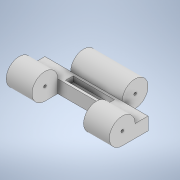
# Autodesk Inventor part: фаланга гусеницы
Saved by Autodesk Inventor 2020.1 (Build 241239000, 239)
## iProperties
Created: 2021-09-27
Part Number: фаланга гусеницы
Material: Типовые
Document SubType Name: Modeling
Designer: User
Density: 1 g/cm^3
Appearance: По умолчанию
Author: User
Autodesk Inventor part; units mm, degrees
ref_plane "YZ Plane" through (0, 0, 0) normal (1, 0, 0) x (0, 1, 0)
ref_plane "XZ Plane" through (0, 0, 0) normal (0, 1, 0) x (-1, 0, 0)
ref_plane "XY Plane" through (0, 0, 0) normal (0, 0, 1) x (1, 0, 0)
sketch "Эскиз1" plane through (0, 0, 0) normal (1, 0, 0) x (0, 1, 0)
  line L0 (0, 0) -> (-5, 0)
  line L1 (-5, 0) -> (-5, -15)
  line L2 (-5, -15) -> (0, -15)
  line L3 (0, -15) -> (0, 0)
  circle A0 centre (0, 0) radius 5
  circle A1 centre (0, -15) radius 5
  circle A2 centre (0, 0) radius 0.5
  circle A3 centre (0, -15) radius 0.5
  point P0 (0, -5)
  point P1 (0, -10)
  dimension "d0" = 5
  dimension "d1" = 15
  dimension "d4" = 1
  dimension "d5" = 1
  constraints: 8 end point, 4 coincident, 2 centre point, 2 parallel, 1 horizontal, 1 perpendicular, 6 other
  measures "d0" distance of L1.end L2.end
  measures "d1" distance of L0.end L1.end
  measures "d4" diameter of A2
  measures "d5" diameter of A3
extrude "Выдавливание1" add sketch "Эскиз1" along normal blind 40 contours A2 L3 A0 L0 | L0 A0 L3 A2 | A0 L3 A1 L1 | A1 L3 A3 L2 | L2 A3 L3 A1
sketch "Эскиз2" plane through (0, 0, -5) normal (0, 1, 0) x (1, 0, 0)
  line L0 (0, 0) -> (40, 0) projected
  line L1 (0, -10) -> (40, -10) projected
  line L2 (10, 0) -> (30, 0)
  line L3 (30, 0) -> (30, -10)
  line L4 (30, -10) -> (10, -10)
  line L5 (10, -10) -> (10, 0)
  line L6 (0, 5) -> (0, 0) projected
  line L7 (40, 5) -> (40, 0) projected
  point P0 (0, -5)
  dimension "d6" = 10
  dimension "d7" = 10
  constraints: 8 end point, 2 parallel, 2 point on line, 1 horizontal, 1 perpendicular
  measures "d6" distance from line of L6 L2.start
  measures "d7" distance from line of L7 L2.end
extrude "Выдавливание2" cut sketch "Эскиз2" along normal mid plane 10
sketch "Эскиз3" plane through (0, 0, -5) normal (0, 1, 0) x (1, 0, 0)
  line L0 (0, 5) -> (40, 5) projected
  line L1 (0, 15) -> (40, 15) projected
  line L2 (10, 5) -> (0, 5)
  line L3 (0, 5) -> (0, 15)
  line L4 (0, 15) -> (10, 15)
  line L5 (10, 15) -> (10, 5)
  line L6 (40, 5) -> (40, 15) projected
  line L7 (30, 5) -> (40, 5)
  line L8 (40, 5) -> (40, 15)
  line L9 (40, 15) -> (30, 15)
  line L10 (30, 15) -> (30, 5)
  line L11 (40, 5) -> (40, 0) projected
  line L12 (0, 5) -> (0, 0) projected
  point P0 (0, -5)
  point P1 (40, 10)
  point P2 (10, 15)
  dimension "d10" = 10
  dimension "d11" = 10
  constraints: 16 end point, 4 parallel, 3 point on line, 2 horizontal, 2 perpendicular
  measures "d10" distance from line of L11 L7.start
  measures "d11" distance from line of L12 L2.start
extrude "Выдавливание3" cut sketch "Эскиз3" against normal mid plane 10 contours L3 L1 L5 L0 | L10 L1 L6 L0
sketch "Эскиз10" plane through (10, 0, -5) normal (0, 1, 0) x (1, 0, 0)
  line L0 (2, 1) -> (18, 1)
  line L1 (18, 1) -> (18, 4)
  line L2 (18, 4) -> (2, 4)
  line L3 (2, 4) -> (2, 1)
  line L4 (20, -10) -> (20, 0) projected
  line L5 (0, 5) -> (0, 15) projected
  line L6 (0, 0) -> (20, 0) projected
  line L7 (-10, 5) -> (0, 5) projected
  point P0 (-10, -5)
  point P1 (20, -5)
  point P2 (0, 10)
  dimension "d37" = 2
  dimension "d38" = 2
  dimension "d39" = 1
  dimension "d40" = 1
  constraints: 8 end point, 2 parallel, 1 horizontal, 1 perpendicular
  measures "d37" distance from line of L4 L0.end
  measures "d38" distance from line of L5 L0.start
  measures "d39" distance from line of L6 L0.start
  measures "d40" distance from line of L7 L2.end
extrude "Выдавливание9" cut sketch "Эскиз10" against normal blind 2
